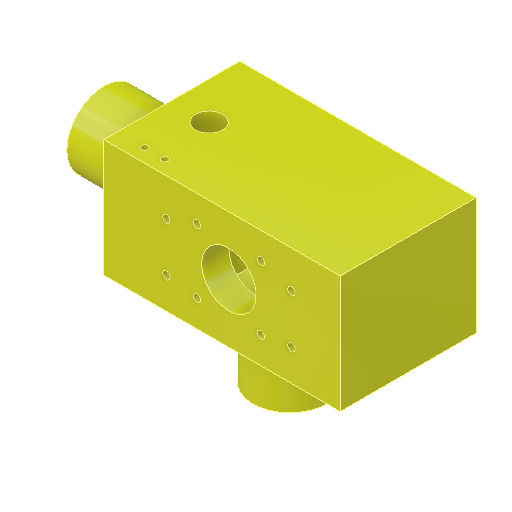
# Autodesk Inventor part: driver_L
Saved by Autodesk Inventor 2022 (Build 260153000, 153)
## iProperties
Created: 2021-04-23
Part Number: driver_L
Material: Generic
Document SubType Name: Modeling
Designer: nnico
Density: 1 g/cm^3
Appearance: Yellow
Author: nnico
Autodesk Inventor part; units mm, degrees
ref_plane "YZ Plane" through (0, 0, 0) normal (1, 0, 0) x (0, 1, 0)
ref_plane "XZ Plane" through (0, 0, 0) normal (0, 1, 0) x (-1, 0, 0)
ref_plane "XY Plane" through (0, 0, 0) normal (0, 0, 1) x (1, 0, 0)
sketch "Sketch1" plane through (0, 0, 0) normal (0, 0, 1) x (1, 0, 0)
  line L0 (-23.55, 23.55) -> (23.55, 23.55) construction
  line L1 (23.55, 23.55) -> (23.55, -23.55) construction
  line L2 (23.55, -23.55) -> (-23.55, -23.55) construction
  line L3 (-23.55, -23.55) -> (-23.55, 23.55) construction
  line L4 (0, 23.55) -> (0, -23.55) construction
  line L5 (-23.55, 0) -> (23.55, 0) construction
  circle A0 centre (-23.55, 23.55) radius 2.75
  circle A1 centre (23.55, 23.55) radius 2.75
  circle A2 centre (-23.55, -23.55) radius 2.75
  circle A3 centre (23.55, -23.55) radius 2.75
  circle A4 centre (0, 0) radius 20
  line L6 (-28.2, 28.2) -> (28.2, 28.2) construction
  line L7 (28.2, 28.2) -> (28.2, -28.2) construction
  line L8 (28.2, -28.2) -> (-28.2, -28.2) construction
  line L9 (-28.2, -28.2) -> (-28.2, 28.2) construction
  line L10 (-28.2, 0) -> (28.2, 0) construction
  line L11 (0, -28.2) -> (0, 28.2) construction
  line L12 (-60, 21.2) -> (-32, 21.2) construction
  line L13 (-32, 21.2) -> (-32, -25.8) construction
  line L14 (-32, -25.8) -> (-60, -25.8) construction
  line L15 (-60, -25.8) -> (-60, 21.2) construction
  line L16 (-46, 21.2) -> (-46, -25.8) construction
  line L17 (-60, -2.3) -> (-32, -2.3) construction
  circle A5 centre (-46, 15.7) radius 2.75
  circle A6 centre (-46, -20.3) radius 2.75
  line L18 (60, 21.2) -> (32, 21.2) construction
  line L19 (32, 21.2) -> (32, -25.8) construction
  line L20 (32, -25.8) -> (60, -25.8) construction
  line L21 (60, -25.8) -> (60, 21.2) construction
  line L22 (46, 21.2) -> (46, -25.8) construction
  line L23 (60, -2.3) -> (32, -2.3) construction
  circle A7 centre (46, 15.7) radius 2.75
  circle A8 centre (46, -20.3) radius 2.75
  line L24 (-82, 43.2) -> (82, 43.2)
  line L25 (82, 43.2) -> (82, -43.2)
  line L26 (82, -43.2) -> (-82, -43.2)
  line L27 (-82, -43.2) -> (-82, 43.2)
  point P0 (0, 0)
  dimension "d0" = 47.1
  dimension "d1" = 47.1
  dimension "d2" = 5.5
  dimension "d4" = 40
  dimension "d5" = 56.4
  dimension "d6" = 56.4
  dimension "d9" = 46
  dimension "d10" = 47
  dimension "d11" = 28
  dimension "d12" = 5.5
  dimension "d13" = 36
  dimension "d14" = 22
  dimension "d15" = 15
  dimension "d18" = 2.3
  constraints: 56 end point, 15 midpoint, 14 symmetric about line, 9 centre point, 8 parallel, 4 horizontal, 4 perpendicular, 3 coincident, 2 point on line, 8 other
  measures "d0" distance of L0.end L1.end
  measures "d1" distance of L0.start L0.end
  measures "d2" diameter of A0
  measures "d4" diameter of A4
  measures "d5" distance of L7.end L8.end
  measures "d6" distance of L6.end L7.end
  measures "d9" horizontal distance of L4.end L16.end
  measures "d10" distance of L14.end L12.start
  measures "d11" distance of L12.start L12.end
  measures "d12" diameter of A5
  measures "d13" diameter of A5.centre L17
  measures "d14" distance between parallel lines of L25 L21
  measures "d15" distance between parallel lines of L24 L6
  measures "d18" distance between parallel lines of L5 L17
extrude "Extrusion1" add sketch "Sketch1" along normal blind 10
sketch "Sketch2" plane through (0, 0, 0) normal (0, 0, -1) x (-1, 0, 0)
  line L0 (32.5, -32.5) -> (-32.5, -32.5)
  line L1 (-32.5, -32.5) -> (-32.5, 32.5)
  line L2 (-32.5, 32.5) -> (32.5, 32.5)
  line L3 (32.5, 32.5) -> (32.5, -32.5)
  line L4 (0, 32.5) -> (0, -32.5) construction
  line L5 (-32.5, 0) -> (32.5, 0) construction
  line L6 (-82, -43.2) -> (-82, 43.2) projected
  line L7 (82, -43.2) -> (-82, -43.2) projected
  line L8 (-82, 43.2) -> (82, 43.2)
  line L9 (82, 43.2) -> (82, -43.2)
  line L10 (82, -43.2) -> (-82, -43.2)
  line L11 (-82, -43.2) -> (-82, 43.2)
  point P0 (0, 0)
  point P1 (0, 0)
  dimension "d19" = 65
  dimension "d20" = 65
  constraints: 20 end point, 5 midpoint, 4 parallel, 2 horizontal, 2 perpendicular, 1 coincident
  measures "d19" distance of L1.end L2.end
  measures "d20" distance of L0.end L1.end
extrude "Extrusion2" add sketch "Sketch2" along normal blind 90
sketch "Sketch3" plane through (0, 0, 0) normal (0, 0, -1) x (-1, 0, 0)
  line L0 (32.5, -32.5) -> (32.5, 32.5) projected
  line L1 (32.5, 32.5) -> (-32.5, 32.5) projected
  line L2 (-32.5, 32.5) -> (-32.5, -32.5) projected
  line L3 (-32.5, -32.5) -> (32.5, -32.5) projected
  circle A0 centre (23.55, 23.55) radius 2.75 projected
  circle A1 centre (-23.55, 23.55) radius 2.75 projected
  circle A2 centre (23.55, -23.55) radius 2.75 projected
  circle A3 centre (-23.55, -23.55) radius 2.75 projected
  circle A4 centre (0, 0) radius 20 projected
extrude "Extrusion3" add sketch "Sketch3" along normal blind 10
sketch "Sketch4" plane through (-82, -43.2, 10) normal (-1, 0, 0) x (0, 0, 1)
  line L0 (0, 0) -> (-100, 0) projected
  line L1 (0, 86.4) -> (0, 0) projected
  line L2 (-100, 86.4) -> (0, 86.4) projected
  line L3 (-100, 0) -> (-100, 86.4) projected
  point P0 (-10, 43.2)
extrude "Extrusion4" add sketch "Sketch4" along normal blind 10
sketch "Sketch5" plane through (82, -43.2, -90) normal (0, -1, 0) x (1, 0, 0)
  line L0 (-174, 0) -> (-174, 100) construction
  line L1 (-174, 50) -> (0, 50) construction
  line L2 (0, 0) -> (0, 100) construction
  line L3 (0, 100) -> (-174, 100) construction
  line L4 (-87, 100) -> (-87, 0) construction
  line L5 (0, 0) -> (-174, 0) construction
  circle A0 centre (-87, 50) radius 27.305
  point P0 (-82, 90)
  dimension "d27" = 54.61
  constraints: 5 midpoint, 4 end point, 1 centre point
  measures "d27" diameter of A0
extrude "Extrusion5" add sketch "Sketch5" along normal blind 50
sketch "Sketch6" plane through (-92, -43.2, 10) normal (-1, 0, 0) x (0, 0, 1)
  line L0 (-100, 75.7) -> (-100, 10.7) construction
  line L1 (-100, 43.2) -> (0, 43.2) construction
  line L2 (0, 0) -> (0, 86.4) construction
  line L3 (-100, 86.4) -> (0, 86.4) construction
  line L4 (-50, 86.4) -> (-50, 0) construction
  line L5 (-100, 0) -> (0, 0) construction
  circle A0 centre (-50, 43.2) radius 27.305
  point P0 (-10, 43.2)
  dimension "d30" = 54.61
  constraints: 5 midpoint, 4 end point, 1 centre point
  measures "d30" diameter of A0
extrude "Extrusion6" add sketch "Sketch6" along normal blind 50
sketch "Sketch7" plane through (-142, 0, -40) normal (-1, 0, 0) x (0, 0, 1)
  circle A0 centre (0, 0) radius 27.305 projected
  circle A1 centre (0, 0) radius 10
  point P0 (40, 0)
  dimension "d33" = 20
  constraints: 1 centre point, 1 coincident
  measures "d33" diameter of A1
extrude "Extrusion7" cut sketch "Sketch7" against normal up to surface (109.5 mm away) contours A1
sketch "Sketch8" plane through (82, 43.2, 10) normal (0, 1, 0) x (1, 0, 0)
  line L0 (-174, 100) -> (-174, 0) construction
  line L1 (-174, 0) -> (-154, 0) construction
  line L2 (-154, 0) -> (-154, 10) construction
  line L3 (-154, 10) -> (-174, 10) construction
  line L4 (-174, 10) -> (-174, 0) construction
  line L5 (0, 0) -> (-174, 0) construction
  line L6 (-154, 10) -> (-139, 10) construction
  line L7 (-139, 10) -> (-139, 0) construction
  line L8 (-139, 0) -> (-154, 0) construction
  line L9 (-154, 0) -> (-154, 10) construction
  circle A0 centre (-139, 10) radius 2.5
  circle A1 centre (-154, 10) radius 2.5
  point P0 (-82, 10)
  dimension "d36" = 20
  dimension "d37" = 10
  dimension "d38" = 15
  dimension "d39" = 5
  dimension "d40" = 5
  constraints: 16 end point, 4 parallel, 2 centre point, 2 coincident, 2 horizontal, 2 perpendicular, 1 point on line
  measures "d36" distance of L3.end L2.end
  measures "d37" distance of L2.end L1.end
  measures "d38" distance of L7.end L8.end
  measures "d39" diameter of A0
  measures "d40" diameter of A1
extrude "Extrusion8" cut sketch "Sketch8" against normal blind 6
sketch "Sketch9" plane through (82, 43.2, 10) normal (0, 1, 0) x (1, 0, 0)
  line L0 (-174, 0) -> (-174, 100) construction
  line L1 (-174, 50) -> (0, 50) construction
  line L2 (0, 100) -> (0, 0) construction
  circle A0 centre (-139, 10) radius 2.5 construction
  circle A1 centre (-154, 10) radius 2.5 construction
  line L3 (-139, 10) -> (-154, 10) construction
  line L4 (-146.5, 10) -> (-146.5, 50) construction
  circle A2 centre (-146.5, 50) radius 10
  point P0 (-82, 10)
  dimension "d43" = 20
  constraints: 6 end point, 3 midpoint, 1 centre point, 1 coincident, 1 horizontal, 1 perpendicular, 1 point on line
  measures "d43" diameter of A2
extrude "Extrusion9" cut sketch "Sketch9" against normal blind 43.2
body "Solid1"
